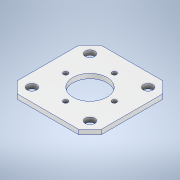
# Autodesk Inventor part: MotorMountingPlate
Saved by Autodesk Inventor 2022 (Build 260153000, 153)
## iProperties
Created: 2021-03-10
Part Number: MotorMountingPlate
Material: Aluminum 6061
Document SubType Name: Modeling
Designer: Esketitttttt
Density: 2.7 g/cm^3
Appearance: Aluminum - Flat
Mass: 75.2816 g
Surface Area: 146.228 cm^2
Volume: 27.8821 cm^3
Author: Esketitttttt
Autodesk Inventor part; units mm, degrees
ref_plane "YZ Plane" through (0, 0, 0) normal (1, 0, 0) x (0, 1, 0)
ref_plane "XZ Plane" through (0, 0, 0) normal (0, 1, 0) x (-1, 0, 0)
ref_plane "XY Plane" through (0, 0, 0) normal (0, 0, 1) x (1, 0, 0)
sketch "Sketch1" plane through (0, 0, 0) normal (0, 1, 0) x (-1, 0, 0)
  circle A0 centre (0, 0) radius 34.925 construction
  circle A1 centre (0, 0) radius 25.019 construction
  line L0 (0, 0) -> (25.019, 0) construction
  line L1 (0, 0) -> (25.019, 0) construction
  line L2 (0, 0) -> (25.019, 0) construction
  circle A2 centre (0, 0) radius 40.64 construction
  circle A3 centre (0, 0) radius 43.18 construction
  circle A4 centre (0, -25.019) radius 2.3813
  circle A5 centre (25.019, 0) radius 2.3813
  circle A6 centre (0, 25.019) radius 2.3813
  circle A7 centre (-25.019, 0) radius 2.3813
  line L3 (-43.18, -43.18) -> (43.18, -43.18)
  line L4 (43.18, -43.18) -> (43.18, 43.18)
  line L5 (43.18, 43.18) -> (-43.18, 43.18)
  line L6 (-43.18, 43.18) -> (-43.18, -43.18)
  line L7 (-43.18, -43.18) -> (43.18, 43.18) construction
  line L8 (43.18, -43.18) -> (-43.18, 43.18) construction
  circle A8 centre (0, 0) radius 6.477
  circle A9 centre (0, 0) radius 17.5768
  point P0 (0, 25.019)
  point P1 (-25.019, 0)
  point P2 (0, -43.18)
  point P3 (0, 0)
  point P4 (0, 0)
  dimension "d6" = 50.038
  dimension "d8" = 360
  dimension "d9" = 2.54
  dimension "d10" = 4.7625
  dimension "d13" = 360
  dimension "d28" = 12.954
  dimension "d29" = 35.1536
  dimension "d33" = 86.36
  dimension "d34" = 86.36
  dimension "d35" = 81.28
  dimension "d36" = 69.85
  constraints: 18 end point, 12 coincident, 10 centre point, 5 midpoint, 3 horizontal, 2 parallel, 2 point on circle, 2 vertical alignment, 1 collinear, 1 perpendicular, 18 other
  measures "d6" diameter of A1
  measures "d9" radial gap between concentric circles of A2 A3
  measures "d10" diameter of A4
  measures "d28" diameter of A8
  measures "d29" diameter of A9
  measures "d33" distance of L5.end L3.start
  measures "d34" distance of L4.end L5.end
  measures "d35" diameter of A2
  measures "d36" diameter of A0
extrude "Extrusion1" add sketch "Sketch1" along normal blind 4.7625 contours L6 L5 L4 L3
sketch "Sketch2" plane through (0, 4.7625, 0) normal (0, 1, 0) x (1, 0, 0)
  circle A0 centre (0, 0) radius 34.925 construction
  line L0 (43.18, 43.18) -> (-43.18, 43.18) construction
  line L1 (-43.18, 43.18) -> (0, 0) construction
  line L2 (-43.18, -43.18) -> (43.18, -43.18) construction
  line L3 (0, 0) -> (43.18, -43.18) construction
  line L4 (43.18, -43.18) -> (43.18, 43.18) construction
  line L5 (43.18, 43.18) -> (0, 0) construction
  line L6 (-43.18, 43.18) -> (-43.18, -43.18) construction
  line L7 (0, 0) -> (-43.18, -43.18) construction
  circle A1 centre (-29.8414, 29.8414) radius 7.2771 construction
  circle A2 centre (-29.8414, -29.8414) radius 7.2771 construction
  circle A3 centre (29.8414, -29.8414) radius 7.2771 construction
  circle A4 centre (29.8414, 29.8414) radius 7.2771 construction
  dimension "d15" = 69.85
  dimension "d16" = 14.5542
  dimension "d19" = 360
  constraints: 8 end point, 5 centre point, 5 coincident, 2 collinear, 2 point on line, 1 perpendicular, 1 tangent, 13 other
  measures "d15" diameter of A0
  measures "d16" diameter of A1
hole "Hole1" at (-29.8414, 4.7625, -29.8414) at (-29.8414, 4.7625, 29.8414) at (29.8414, 4.7625, 29.8414) at (29.8414, 4.7625, -29.8414) direction (0, -1, 0) diameter 9.779 depth 27.0002
chamfer "Chamfer1" distance 11.43 angle 45 4 edges at (-43.18, 2.3813, 43.18) (43.18, 2.3813, 43.18) (43.18, 2.3813, -43.18) (-43.18, 2.3813, -43.18)
body "Solid1"
